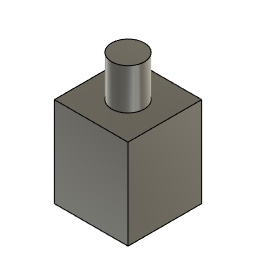
ButtonCap (Autodesk Fusion 360 design; units mm, degrees)
Autodesk Fusion 360 part; units mm, degrees
sketch "Sketch1" plane through (0, 0, 0) normal (0, 1, 0) x (1, 0, 0) in component "RectangleBaseCap"
  line L0 (8.6959, 0, -1.1385) -> (17.6959, 0, -1.1385)
  line L1 (17.6959, 0, -1.1385) -> (17.6959, 0, 7.8615)
  line L2 (17.6959, 0, 7.8615) -> (8.6959, 0, 7.8615)
  line L3 (8.6959, 0, 7.8615) -> (8.6959, 0, -1.1385)
  dimension "d21" = 9
  dimension "d22" = 9
extrude "Extrude1" add sketch "Sketch1" against normal blind 7 contours L0 L1 L2 L3 in plane through (0, 0, 0) normal (0, 0, -1) in component "RectangleBaseCap"
sketch "Sketch2" plane through (0, 0, 7) normal (0, 0, 1) x (-1, 0, 0) in component "RectangleBaseCap"
  line L0 (-8.6959, -7.8615) -> (-8.6959, 1.1385)
  line L1 (-8.6959, 1.1385) -> (-17.6959, 1.1385)
  line L2 (-17.6959, 1.1385) -> (-17.6959, -7.8615)
  line L3 (-17.6959, -7.8615) -> (-8.6959, -7.8615)
  circle A0 centre (-13.1959, -3.3615) radius 2
  dimension "d25" = 4
  measures "d25" diameter of A0
extrude "Extrude2" add sketch "Sketch2" along normal blind 5 contours A0 in component "RectangleBaseCap"
move_body "Move1" [no effect]
extrude "Extrude3" add 1 faces at (11.6959, 1.8615, 0) along direction (0, 0, -1) blind 4 in component "RectangleBaseCap"
sketch "Sketch3" plane through (0, 0, -4) normal (0, 0, -1) x (1, 0, 0) in component "RectangleBaseCap"
  line L0 (8.6959, 1.1385) -> (8.6959, -7.8615)
  line L1 (8.6959, -7.8615) -> (17.6959, -7.8615)
  line L2 (17.6959, -7.8615) -> (17.6959, 1.1385)
  line L3 (17.6959, 1.1385) -> (8.6959, 1.1385)
  line L4 (9.2959, -7.2615) -> (17.0959, -7.2615)
  line L5 (17.0959, -7.2615) -> (17.0959, 0.5385)
  line L6 (17.0959, 0.5385) -> (9.2959, 0.5385)
  line L7 (9.2959, 0.5385) -> (9.2959, -7.2615)
  line L8 (8.6959, -3.3615) -> (9.2959, -3.3615) construction
  line L9 (13.1959, -7.8615) -> (13.1959, -7.2615) construction
  dimension "d30" = 7.8
  dimension "d31" = 7.8
  constraint horizontal L4
  constraint vertical L5
  constraint horizontal L6
  constraint vertical L7
  constraint midpoint L0 L8.start
  constraint midpoint L7 L8.end
  constraint perpendicular L0 L8
  constraint midpoint L1 L9.start
  constraint midpoint L4 L9.end
  constraint perpendicular L1 L9
  measures "d30" distance of L4.start L6.end
  measures "d31" distance of L5 L7
extrude "Extrude4" cut sketch "Sketch3" against normal blind 4 contours L4 L5 L6 L7 in component "RectangleBaseCap"
component "RectangleBaseCap" placed x (1, 0, 0) y (0, 1, 0) z (0, 0, 1) at (0, 0, 0)
equation "CapWidth = 9 mm"
equation "CapHeight = 7 mm"
equation "topDiameter = 4 mm"
equation "topHeight = 5 mm"
equation "buttonWidth = 7.8 mm"
equation "buttonHeight = 4 mm"
equation "d21 = CapWidth"
equation "d22 = CapWidth"
equation "d23 = CapHeight"
equation "d25 = topDiameter"
equation "d26 = topHeight"
equation "d28 = buttonHeight"
equation "d30 = buttonWidth"
equation "d31 = buttonWidth"
equation "d34 = -buttonHeight"
